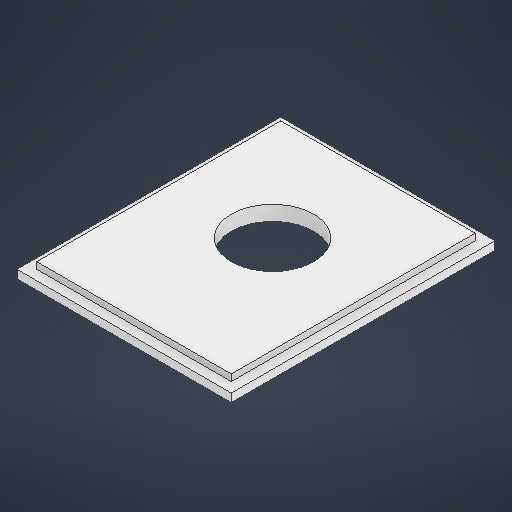
# Autodesk Inventor part: OGRobotRoof
Saved by Autodesk Inventor 2027 (Build 310192060, 192F)
## iProperties
Created: 2026-07-04
Part Number: OGRobotRoof
Material: ABS Plastic
Document SubType Name: Modeling
Designer: machnach0
Density: 1.06 g/cm^3
Appearance: Smooth - White
Author: machnach0
Autodesk Inventor part; units mm, degrees
ref_plane "YZ Plane" through (0, 0, 0) normal (1, 0, 0) x (0, 1, 0)
ref_plane "XZ Plane" through (0, 0, 0) normal (0, 1, 0) x (-1, 0, 0)
ref_plane "XY Plane" through (0, 0, 0) normal (0, 0, 1) x (1, 0, 0)
sketch "Sketch1" plane through (0, 0, 0) normal (0, 1, 0) x (-1, 0, 0)
  line L0 (0, 0) -> (165.1, 0)
  line L1 (165.1, 0) -> (165.1, -203.2)
  line L2 (165.1, -203.2) -> (0, -203.2)
  line L3 (0, -203.2) -> (0, 0)
  line L4 (157.48, -195.58) -> (157.48, -7.62)
  line L5 (157.48, -7.62) -> (7.62, -7.62)
  line L6 (7.62, -7.62) -> (7.62, -195.58)
  line L7 (7.62, -195.58) -> (157.48, -195.58)
  circle A0 centre (82.55, -114.3) radius 31.75
  point P0 (82.55, -195.58)
  point P1 (157.48, -114.3)
  dimension "d0" = 203.2
  dimension "d1" = 165.1
  dimension "d2" = 7.62
  dimension "d3" = 63.5
  dimension "d4" = 88.9
  constraints: 16 end point, 4 parallel, 2 perpendicular, 1 centre point, 1 horizontal, 1 horizontal alignment, 1 midpoint, 1 point on line, 1 vertical alignment, 3 other
  measures "d0" distance of L0.end L1.end
  measures "d1" distance of L1.end L2.end
  measures "d2" distance between parallel lines of L2 L7
  measures "d3" diameter of A0
  measures "d4" distance from line of L2 point (157.48, -114.3)
extrude "Extrusion1" add sketch "Sketch1" along normal blind 6.35 contours L0 L1 L2 L3 | L7 L6 L5 L4 | A0
extrude "Extrusion2" add sketch "Sketch1" along normal blind 11.43 contours L7 L6 L5 L4
extrude "Extrusion3" cut sketch "Sketch1" along normal through all contours A0
body "Solid1"
